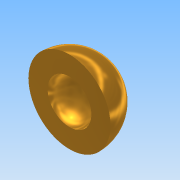
# Autodesk Inventor part: Ball_Half Sphere 3
Saved by Autodesk Inventor 2018.1 (Build 221171000, 171)
## iProperties
Created: 2019-02-18
Part Number: Ball_Half Sphere 3
Material: Nylon 6/6
Document SubType Name: Modeling
Designer: James
Density: 1.13 g/cm^3
Appearance: Metal 1800F Hot
Author: James
Autodesk Inventor part; units mm, degrees
ref_plane "YZ Plane" through (0, 0, 0) normal (1, 0, 0) x (0, 1, 0)
ref_plane "XZ Plane" through (0, 0, 0) normal (0, 1, 0) x (-1, 0, 0)
ref_plane "XY Plane" through (0, 0, 0) normal (0, 0, 1) x (1, 0, 0)
sketch "Sketch1" plane through (0, 0, 0) normal (0, 0, 1) x (1, 0, 0)
  line L0 (0, 0) -> (0, 15)
  line L1 (0, 0) -> (15, 0)
  arc A0 (15, 0) -> (0, 15) centre (0, 0) ccw
  line L2 (0, -3.6213) -> (0, 21.7279) projected
  dimension "d2" = 15
  constraints: 4 end point, 2 coincident, 2 point on circle, 1 centre point, 1 horizontal, 1 vertical
  measures "d2" distance of L0.start L0.end
revolve "Revolution1" add sketch "Sketch1" angle 360 about axis through (0, -10, 0) along (0, 1, 0)
shell "Shell2" thickness 7 removed faces 1 at (4.7094, 0, 0)
body "Solid1"
